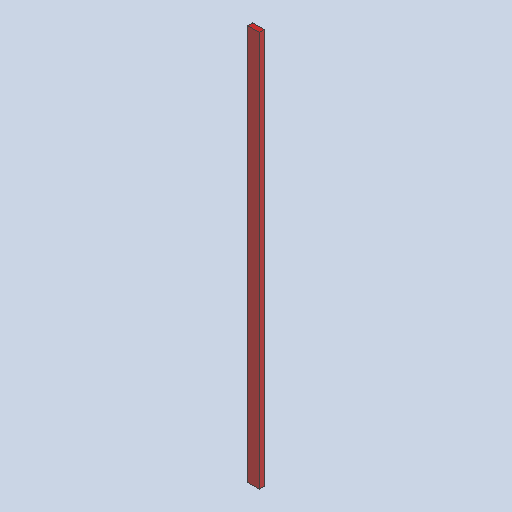
# Autodesk Inventor part: 10'x2x4
Saved by Autodesk Inventor 2025 (Build 290162000, 162)
## iProperties
Created: 2024-09-16
Part Number: 10'x2x4
Material: Generic
Document SubType Name: Modeling
Designer: User
Density: 1 g/cm^3
Appearance: Default
Stock Number: 8
Finish1_Area: 1210.500 in^2
Finish1_Appearance: Red
Finish1_Process: Prime/Paint RAL 3018
Finish1_Description: Prime/Paint RAL 3018
Finish1_ShortDescription: RAL 3018
Finish1_Thickness: 0.002 in
Author: User
Autodesk Inventor part; units mm, degrees
ref_plane "YZ Plane" through (0, 0, 0) normal (1, 0, 0) x (0, 1, 0)
ref_plane "XZ Plane" through (0, 0, 0) normal (0, 1, 0) x (-1, 0, 0)
ref_plane "XY Plane" through (0, 0, 0) normal (0, 0, 1) x (1, 0, 0)
sketch "Sketch1" plane through (0, 0, 0) normal (0, 1, 0) x (-1, 0, 0)
  line L0 (-44.45, -19.05) -> (44.45, -19.05)
  line L1 (44.45, -19.05) -> (44.45, 19.05)
  line L2 (44.45, 19.05) -> (-44.45, 19.05)
  line L3 (-44.45, 19.05) -> (-44.45, -19.05)
  line L4 (-44.45, -19.05) -> (44.45, 19.05) construction
  line L5 (44.45, -19.05) -> (-44.45, 19.05) construction
  point P0 (0, 0)
  dimension "d0" = 38.1
  dimension "d1" = 88.9
  constraints: 12 end point, 2 midpoint, 2 parallel, 1 horizontal, 1 perpendicular
  measures "d0" distance of L0.end L1.end
  measures "d1" distance of L1.end L2.end
extrude "Extrusion1" add sketch "Sketch1" along normal blind 3048
body "Solid1"
